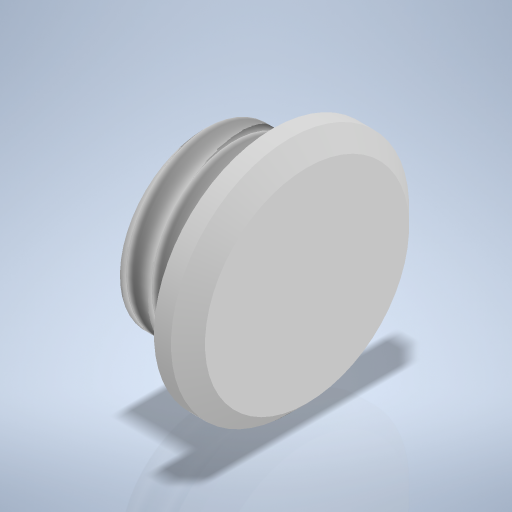
# Autodesk Inventor part: 1072
Saved by Autodesk Inventor 2024 (Build 280153000, 153)
## iProperties
Created: 2024-06-07
Part Number: 1072
Material: Generisch
Document SubType Name: Modeling
Designer: ffogue
Density: 1 g/cm^3
Appearance: Vorgabe
Author: ffogue
Autodesk Inventor part; units mm, degrees
ref_plane "YZ Plane" through (0, 0, 0) normal (1, 0, 0) x (0, 1, 0)
ref_plane "XZ Plane" through (0, 0, 0) normal (0, 1, 0) x (-1, 0, 0)
ref_plane "XY Plane" through (0, 0, 0) normal (0, 0, 1) x (1, 0, 0)
sketch "Skizze1" plane through (0, 0, 0) normal (0, 1, 0) x (-1, 0, 0)
  line L0 (0, 0) -> (0, 5)
  line L1 (0, 5) -> (-4, 5)
  line L2 (-4, 5) -> (-4, 7)
  line L3 (-4, 7) -> (-6, 7)
  line L4 (-6, 7) -> (-6, 0)
  line L5 (-6, 0) -> (0, 0)
  dimension "d0" = 14
  dimension "d1" = 10
  dimension "d2" = 2
  dimension "d3" = 4
  constraints: 12 end point, 5 perpendicular, 1 vertical
  measures "d0" diameter of L3 L5
  measures "d1" diameter of L1 L5
  measures "d2" distance of L2.end L3.end
  measures "d3" distance between parallel lines of L2 L0
revolve "Umdrehung1" add sketch "Skizze1" angle 360 about axis through (6, 0, 0) along (-1, 0, 0)
chamfer "Fasen1" distance 1 angle 45 1 edges at (6, 0, -7)
thread "Gewinde1" size "M10x1.5" class "6g" standard "ISO Metric profile" length 4
